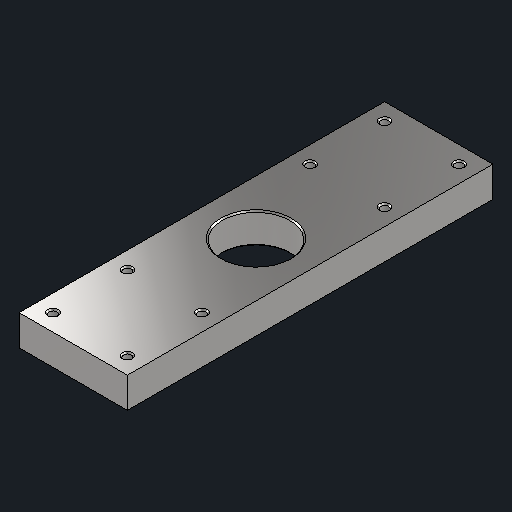
# Autodesk Inventor part: KN-00-02-01
Saved by Autodesk Inventor 2025.2 (Build 292293000, 293)
## iProperties
Created: 2025-03-24
Part Number: KN-00-02-01
Material: X5CrNi18-10
Document SubType Name: Modeling
Designer: Kacper Mik
Density: 8 g/cm^3
Appearance: Semi-Polished
Mass: 31.4003 g
Surface Area: 26.9422 cm^2
Volume: 3.92503 cm^3
Author: Kacper Mik
Autodesk Inventor part; units mm, degrees
ref_plane "YZ Plane" through (0, 0, 0) normal (1, 0, 0) x (0, 1, 0)
ref_plane "XZ Plane" through (0, 0, 0) normal (0, 1, 0) x (-1, 0, 0)
ref_plane "XY Plane" through (0, 0, 0) normal (0, 0, 1) x (1, 0, 0)
sketch "Sketch1" plane through (0, 0, 0) normal (0, 1, 0) x (-1, 0, 0)
  line L0 (0, 0) -> (16, 0)
  line L1 (16, 0) -> (16, -54)
  line L2 (16, -54) -> (0, -54)
  line L3 (0, -54) -> (0, 0)
  dimension "d0" = 16
  dimension "d1" = 54
  constraints: 8 end point, 2 parallel, 1 horizontal, 1 perpendicular
  measures "d0" distance of L1.end L2.end
  measures "d1" distance of L0.end L1.end
extrude "Extrusion1" add sketch "Sketch1" along normal blind 4.5
sketch "Sketch2" plane through (0, 4.5, 0) normal (0, 1, 0) x (1, 0, 0)
  line L0 (-16, 0) -> (0, 0) projected
  line L1 (0, 0) -> (0, 54) projected
  line L2 (0, 54) -> (-16, 54) projected
  line L3 (-16, 54) -> (-16, 0) projected
  line L4 (-16, 0) -> (0, 0) projected
  line L5 (0, 0) -> (0, 54) projected
  line L6 (-16, 0) -> (0, 54) construction
  line L7 (-16, 54) -> (-16, 0) construction
  line L8 (-16, 54) -> (0, 0) construction
  point P0 (-8, 27)
  point P1 (-8, 27)
  constraints: 4 end point, 1 coincident, 1 midpoint
hole "Hole1" at (-8, 4.5, -27) direction (0, -1, 0) diameter 10 end through all
chamfer "Chamfer1" distance 0.2 angle 45 2 edges at (-8, 0, -32) (-8, 4.5, -32)
sketch "Sketch3" plane through (0, 4.5, 0) normal (0, 1, 0) x (1, 0, 0)
  line L0 (0, 38) -> (-16, 38) construction
  line L1 (-16, 38) -> (-16, 54) construction
  line L2 (-16, 54) -> (0, 54) construction
  line L3 (0, 54) -> (0, 38) construction
  line L4 (0, 38) -> (-16, 54) construction
  line L5 (-16, 38) -> (0, 54) construction
  line L6 (-2.5, 51.5) -> (-13.5, 51.5) construction
  line L7 (-13.5, 51.5) -> (-13.5, 40.5) construction
  line L8 (-13.5, 40.5) -> (-2.5, 40.5) construction
  line L9 (-2.5, 40.5) -> (-2.5, 51.5) construction
  line L10 (-2.5, 51.5) -> (-13.5, 40.5) construction
  line L11 (-13.5, 51.5) -> (-2.5, 40.5) construction
  line L12 (0, 54) -> (-16, 54) construction
  line L13 (-16, 54) -> (-16, 0) construction
  line L14 (-16, 0) -> (0, 0) construction
  line L15 (0, 0) -> (0, 54) construction
  circle A0 centre (-8, 27) radius 5.2 construction
  line L16 (-16, 27) -> (0, 27) construction
  point P0 (-8, 46)
  point P1 (-2.5, 13.5)
  point P2 (-13.5, 13.5)
  point P3 (-13.5, 2.5)
  point P4 (-2.5, 2.5)
  dimension "d16" = 16
  dimension "d17" = 16
  dimension "d18" = 11
  dimension "d19" = 11
  constraints: 26 end point, 6 midpoint, 5 coincident, 4 parallel, 4 symmetric about line, 2 horizontal, 2 perpendicular
  measures "d16" distance of L1.end L2.end
  measures "d17" distance of L0.end L1.end
  measures "d18" distance of L8.end L7.end
  measures "d19" distance of L7.end L6.end
hole "Hole2" at (-2.5, 4.5, -40.5) at (-13.5, 4.5, -40.5) at (-13.5, 4.5, -51.5) at (-2.5, 4.5, -51.5) at (-13.5, 4.5, -2.5) at (-13.5, 4.5, -13.5) at (-2.5, 4.5, -13.5) at (-2.5, 4.5, -2.5) direction (0, -1, 0) diameter 1.1835 end through all thread size "M1.4x0.3" class "6H" standard "ISO Metric profile"
chamfer "Chamfer2" distance 0.2 angle 45 8 edges at (-2.5, 4.5, -52.0917) (-2.5, 4.5, -41.0917) (-13.5, 4.5, -52.0917) (-13.5, 4.5, -41.0917) (-2.5, 4.5, -14.0917) (-2.5, 4.5, -3.0917) (-13.5, 4.5, -14.0917) (-13.5, 4.5, -3.0917)
body "Solid1"
